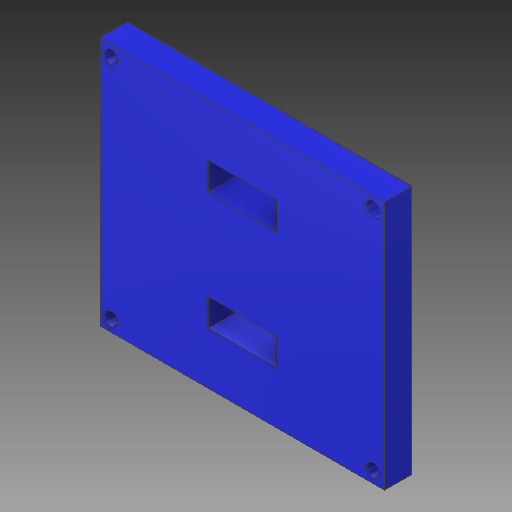
# Autodesk Inventor part: support_card
Saved by Autodesk Inventor 2019 (Build 230136000, 136)
## iProperties
Created: 2018-09-21
Part Number: support_card
Material: Générique
Document SubType Name: Modeling
Designer: Jérémy
Density: 1 g/cm^3
Appearance: Par défaut
Author: Jérémy
Autodesk Inventor part; units mm, degrees
ref_plane "YZ Plane" through (0, 0, 0) normal (1, 0, 0) x (0, 1, 0)
ref_plane "XZ Plane" through (0, 0, 0) normal (0, 1, 0) x (-1, 0, 0)
ref_plane "XY Plane" through (0, 0, 0) normal (0, 0, 1) x (1, 0, 0)
sketch "Esquisse1" plane through (0, 0, 0) normal (0, 0, 1) x (1, 0, 0)
  circle A0 centre (28.6, 24.9) radius 1.5 projected
  circle A1 centre (28.6, -24.78) radius 1.5 projected
  circle A2 centre (-28.75, 24.9) radius 1.5 projected
  circle A3 centre (-28.75, -24.78) radius 1.5 projected
  line L0 (31.1, 27.4) -> (-31.25, 27.4) projected
  line L1 (-31.25, 27.4) -> (-31.25, -27.28) projected
  line L2 (-31.25, -27.28) -> (31.1, -27.28) projected
  line L3 (31.1, -27.28) -> (31.1, 27.4) projected
  line L4 (-7.575, 16) -> (-0.075, 16)
  line L5 (-0.075, 16) -> (7.425, 16)
  line L6 (7.425, 16) -> (7.425, 10)
  line L7 (7.425, 10) -> (-0.075, 10)
  line L8 (-0.075, 10) -> (-7.575, 10)
  line L9 (-7.575, 10) -> (-7.575, 16)
  line L10 (-0.075, 37.051) -> (-0.075, -38.1524) construction
  line L11 (34.7968, 0.06) -> (-21.7073, 0.06) construction
  line L12 (-7.575, -15.88) -> (-0.075, -15.88)
  line L13 (-0.075, -15.88) -> (7.425, -15.88)
  line L14 (7.425, -15.88) -> (7.425, -9.88)
  line L15 (7.425, -9.88) -> (-0.075, -9.88)
  line L16 (-0.075, -9.88) -> (-7.575, -9.88)
  line L17 (-7.575, -9.88) -> (-7.575, -15.88)
  line L18 (-0.075, -36.931) -> (-0.075, 38.2724) construction
  point P0 (0, 0)
  point P1 (-0.075, 27.4)
  point P2 (31.1, 0.06)
  dimension "d0" = 7.5
  dimension "d1" = 16
  dimension "d2" = 6
  constraints: 30 end point, 8 point on line, 8 symmetric about line, 3 perpendicular, 2 collinear, 2 horizontal, 2 midpoint, 1 vertical
  measures "d0" distance of L4.end L5.end
  measures "d1" vertical distance of L5.end point (0, 0)
  measures "d2" distance of L5.end L6.end
extrude "Extrusion1" add sketch "Esquisse1" along normal blind 6
equation "\"d0\" = 0.5 * L_attache_carte"
equation "\"d1\" = 0.5 * largeur"
equation "\"d2\" = epaisseur"
equation "\"d3\" = epaisseur"
equation "\"epaisseur\" = 6"
equation "\"ecartement\" = 25"
equation "\"dvis\" = 3"
equation "\"largeur\" = 32"
equation "\"L_attache_carte\" = 15"
equation "\"marge_attache_carte\" = 5"
equation "\"L_cubi\" = 81.6"
equation "\"taille_trou\" = 7"
equation "\"L_moteur\" = 28.3"
equation "\"marge_trou\" = 2"
equation "\"largeur_cubi\" = 81.6"
equation "\"H_cubi\" = 81.6"
equation "\"epaisseur_wheel\" = 9"
equation "\"H_nez\" = 25"
equation "\"chanfrein\" = 0.5"
equation "\"H_trou_int\" = 0.2"
equation "\"L_trou_int\" = 1"
equation "\"pos_trou_int_1\" = 0.7"
equation "\"pos_trou_int_2\" = 3"
equation "\"epaisseur_metabois\" = 3"
equation "\"L_metabois\" = 8.2"
equation "\"epaisseur_modules\" = 6"
